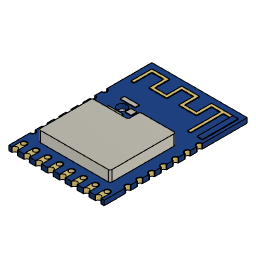
EMB1061_BLE4.2_BlueNRG-132 v2 (Autodesk Fusion 360 design; units mm, degrees)
Autodesk Fusion 360 part; units mm, degrees
sketch "Sketch1" plane through (0, 0, 0) normal (0, 0, 1) x (1, 0, 0)
  line L0 (16, 24) -> (0, 24)
  line L1 (1.5, 1.5) -> (1.5, 0)
  line L2 (0.5, 0) -> (0.5, 1.5)
  arc A0 (1.45, 0) -> (0.55, 0) centre (1, 0) ccw
  line L3 (2.5, 0) -> (2.5, 1.5)
  line L4 (3.5, 1.5) -> (3.5, 0)
  line L5 (3.5, 0) -> (3.45, 0)
  circle A1 centre (3, 1.5) radius 0.4
  arc A2 (3.45, 0) -> (2.55, 0) centre (3, 0) ccw
  line L6 (4.5, 0) -> (4.5, 1.5)
  line L7 (5.5, 1.5) -> (5.5, 0)
  circle A3 centre (5, 1.5) radius 0.4
  arc A4 (5.45, 0) -> (4.55, 0) centre (5, 0) ccw
  line L8 (6.5, 0) -> (6.5, 1.5)
  line L9 (7.5, 1.5) -> (7.5, 0)
  circle A5 centre (7, 1.5) radius 0.4
  arc A6 (7.45, 0) -> (6.55, 0) centre (7, 0) ccw
  line L10 (0.5, 0) -> (0.5, 1.5)
  line L11 (1.5, 1.5) -> (1.5, 0)
  circle A7 centre (1, 1.5) radius 0.4
  arc A8 (1.45, 0) -> (0.55, 0) centre (1, 0) ccw
  line L12 (9.5, 1.5) -> (9.5, 0)
  arc A9 (9.45, 0) -> (8.55, 0) centre (9, 0) ccw
  line L13 (8.5, 0) -> (8.5, 1.5)
  circle A10 centre (9, 1.5) radius 0.4
  line L14 (11.5, 1.5) -> (11.5, 0)
  arc A11 (11.45, 0) -> (10.55, 0) centre (11, 0) ccw
  line L15 (10.5, 0) -> (10.5, 1.5)
  circle A12 centre (11, 1.5) radius 0.4
  line L16 (13.5, 1.5) -> (13.5, 0)
  arc A13 (13.45, 0) -> (12.55, 0) centre (13, 0) ccw
  line L17 (12.5, 0) -> (12.5, 1.5)
  circle A14 centre (13, 1.5) radius 0.4
  line L18 (15.5, 1.5) -> (15.5, 0)
  arc A15 (15.45, 0) -> (14.55, 0) centre (15, 0) ccw
  line L19 (14.5, 0) -> (14.5, 1.5)
  circle A16 centre (15, 1.5) radius 0.4
  line L20 (1.5, 0) -> (1.45, 0)
  line L21 (0.55, 0) -> (0.5, 0)
  line L22 (1.5, 0) -> (1.45, 0)
  line L23 (0.55, 0) -> (0.5, 0)
  line L24 (5.5, 0) -> (5.45, 0)
  line L25 (4.55, 0) -> (4.5, 0)
  line L26 (3.45, 0) -> (4.55, 0)
  line L27 (7.5, 0) -> (7.45, 0)
  line L28 (6.55, 0) -> (6.5, 0)
  line L29 (5.45, 0) -> (6.55, 0)
  line L30 (7.45, 0) -> (8.55, 0)
  line L31 (9.45, 0) -> (10.55, 0)
  line L32 (11.45, 0) -> (12.55, 0)
  line L33 (13.45, 0) -> (14.55, 0)
  line L34 (15.45, 0) -> (16, 0)
  arc A17 (0, 3.6) -> (0, 4.4) centre (0, 4) ccw
  arc A18 (0, 5.6) -> (0, 6.4) centre (0, 6) ccw
  arc A19 (0, 7.6) -> (0, 8.4) centre (0, 8) ccw
  arc A20 (0, 9.6) -> (0, 10.4) centre (0, 10) ccw
  arc A21 (0, 11.6) -> (0, 12.4) centre (0, 12) ccw
  arc A22 (0, 13.6) -> (0, 14.4) centre (0, 14) ccw
  arc A23 (0, 15.6) -> (0, 16.4) centre (0, 16) ccw
  arc A24 (16, 6.4) -> (16, 5.6) centre (16, 6) ccw
  arc A25 (16, 16.4) -> (16, 15.6) centre (16, 16) ccw
  arc A26 (16, 4.4) -> (16, 3.6) centre (16, 4) ccw
  arc A27 (16, 10.4) -> (16, 9.6) centre (16, 10) ccw
  arc A28 (16, 8.4) -> (16, 7.6) centre (16, 8) ccw
  arc A29 (16, 14.4) -> (16, 13.6) centre (16, 14) ccw
  arc A30 (16, 12.4) -> (16, 11.6) centre (16, 12) ccw
  line L35 (0, 24) -> (0, 16.4)
  line L36 (0, 15.6) -> (0, 14.4)
  line L37 (0, 13.6) -> (0, 12.4)
  line L38 (0, 11.6) -> (0, 10.4)
  line L39 (0, 9.6) -> (0, 8.4)
  line L40 (0, 7.6) -> (0, 6.4)
  line L41 (0, 5.6) -> (0, 4.4)
  line L42 (0, 3.6) -> (0, 0)
  line L43 (0, 3.5) -> (0, 3.6)
  line L44 (0, 4.4) -> (0, 4.5)
  line L45 (16, 0) -> (16, 3.6)
  line L46 (16, 4.4) -> (16, 5.6)
  line L47 (16, 6.4) -> (16, 7.6)
  line L48 (16, 8.4) -> (16, 9.6)
  line L49 (16, 10.4) -> (16, 11.6)
  line L50 (16, 12.4) -> (16, 13.6)
  line L51 (16, 14.4) -> (16, 15.6)
  line L52 (16, 16.4) -> (16, 24)
  arc A31 (1.5, 1.5) -> (0.5, 1.5) centre (1, 1.5) ccw
  arc A32 (3.5, 1.5) -> (2.5, 1.5) centre (3, 1.5) ccw
  arc A33 (0, 3.5) -> (0, 4.5) centre (0, 4) ccw
  arc A34 (0, 5.5) -> (0, 6.5) centre (0, 6) ccw
  arc A35 (0, 7.5) -> (0, 8.5) centre (0, 8) ccw
  arc A36 (0, 9.5) -> (0, 10.5) centre (0, 10) ccw
  arc A37 (0, 11.5) -> (0, 12.5) centre (0, 12) ccw
  arc A38 (0, 13.5) -> (0, 14.5) centre (0, 14) ccw
  arc A39 (16, 16.5) -> (16, 15.5) centre (16, 16) ccw
  arc A40 (16, 14.5) -> (16, 13.5) centre (16, 14) ccw
  arc A41 (16, 12.5) -> (16, 11.5) centre (16, 12) ccw
  arc A42 (16, 10.5) -> (16, 9.5) centre (16, 10) ccw
  arc A43 (16, 6.5) -> (16, 5.5) centre (16, 6) ccw
  arc A44 (16, 4.5) -> (16, 3.5) centre (16, 4) ccw
  arc A45 (16, 8.5) -> (16, 7.5) centre (16, 8) ccw
  arc A46 (0, 15.5) -> (0, 16.5) centre (0, 16) ccw
  arc A47 (7.5, 1.5) -> (6.5, 1.5) centre (7, 1.5) ccw
  arc A48 (5.5, 1.5) -> (4.5, 1.5) centre (5, 1.5) ccw
  arc A49 (9.5, 1.5) -> (8.5, 1.5) centre (9, 1.5) ccw
  arc A50 (11.5, 1.5) -> (10.5, 1.5) centre (11, 1.5) ccw
  arc A51 (13.5, 1.5) -> (12.5, 1.5) centre (13, 1.5) ccw
  arc A52 (15.5, 1.5) -> (14.5, 1.5) centre (15, 1.5) ccw
  line L53 (0, 0) -> (0.55, 0)
  line L54 (1.45, 0) -> (2.55, 0)
  line L55 (13.5, 17) -> (13, 17)
  line L56 (13, 17) -> (13, 22.5)
  line L57 (13.5, 22.5) -> (13.5, 17)
  line L58 (1.5, 22.5) -> (1.5, 19.5)
  line L59 (1.5, 19.5) -> (1, 19.5)
  line L60 (1, 19.5) -> (1, 23)
  line L61 (1, 23) -> (4, 23)
  line L62 (4, 23) -> (4, 20.5)
  line L63 (3.5, 20) -> (3.5, 22.5)
  line L64 (4, 20.5) -> (6, 20.5)
  line L65 (6.5, 20) -> (3.5, 20)
  line L66 (6, 20.5) -> (6, 23)
  line L67 (6.5, 22.5) -> (6.5, 20)
  line L68 (9, 20.5) -> (11, 20.5)
  line L69 (8.5, 20) -> (8.5, 22.5)
  line L70 (9, 23) -> (9, 20.5)
  line L71 (8.5, 20) -> (11.5, 20)
  line L72 (11.5, 20) -> (11.5, 22.5)
  line L73 (11, 23) -> (11, 20.5)
  line L74 (14.6, 23) -> (11, 23)
  line L75 (11.5, 22.5) -> (13, 22.5)
  line L76 (9, 23) -> (6, 23)
  line L77 (1.5, 22.5) -> (3.5, 22.5)
  line L78 (6.5, 22.5) -> (8.5, 22.5)
  line L79 (13.5, 22.5) -> (14.6, 22.5)
  line L80 (14.6, 22.5) -> (14.6, 23)
  line L81 (2.3, 3) -> (13.7, 3)
  line L82 (14, 3.3) -> (14, 13.7)
  line L83 (13.7, 14) -> (8.3, 14)
  line L84 (2, 11.7) -> (2, 3.3)
  line L85 (2.3, 12) -> (7.7, 12)
  line L86 (8, 12.3) -> (8, 13.7)
  circle A53 centre (4, 15) radius 0.8
  line L87 (2.7, 16.7) -> (5.2, 16.7)
  line L88 (5.2, 16.7) -> (5.2, 16)
  line L89 (5.2, 16) -> (2.7, 16)
  line L90 (2.7, 16) -> (2.7, 16.7)
  line L91 (2.7, 14) -> (5.2, 14)
  line L92 (5.2, 14) -> (5.2, 13.3)
  line L93 (5.2, 13.3) -> (2.7, 13.3)
  line L94 (2.7, 13.3) -> (2.7, 14)
  line L95 (5, 15.5) -> (6, 15.5)
  line L96 (6, 15.5) -> (6, 14.5)
  line L97 (6, 14.5) -> (5, 14.5)
  line L98 (5, 14.5) -> (5, 15.5)
  arc A54 (8.3, 14) -> (8, 13.7) centre (8.3, 13.7) ccw
  arc A55 (14, 13.7) -> (13.7, 14) centre (13.7, 13.7) ccw
  arc A56 (13.7, 3) -> (14, 3.3) centre (13.7, 3.3) ccw
  arc A57 (2, 3.3) -> (2.3, 3) centre (2.3, 3.3) ccw
  arc A58 (2.3, 12) -> (2, 11.7) centre (2.3, 11.7) ccw
  arc A59 (7.7, 12) -> (8, 12.3) centre (7.7, 12.3) ccw
  line L99 (15.5, 23) -> (14.602, 23)
  line L100 (14.602, 23) -> (14.602, 17)
  line L101 (14.602, 17) -> (15.5, 17)
  line L102 (15.5, 17) -> (15.5, 23)
  dimension "d1" = 16
  dimension "d2" = 24
  dimension "d23" = 0.8
  dimension "d24" = 0.8
  dimension "d25" = 0.8
  dimension "d26" = 0.8
  dimension "d27" = 0.8
  dimension "d28" = 0.8
  dimension "d29" = 0.8
  dimension "d30" = 0.8
  dimension "d31" = 0.4
  dimension "d32" = 0.4
  dimension "d33" = 0.4
  dimension "d34" = 0.4
  dimension "d35" = 0.4
  dimension "d36" = 0.4
  dimension "d37" = 0.4
  dimension "d38" = 0.4
  dimension "d39" = 0.4
  dimension "d40" = 0.4
  dimension "d41" = 0.4
  dimension "d42" = 0.4
  dimension "d43" = 0.4
  dimension "d44" = 0.4
  dimension "d54" = 0.3
  constraint horizontal L53
  constraint vertical L45
  constraint horizontal L0
  constraint vertical L35
  constraint coincident L42.end L53.start
  constraint vertical L1
  constraint horizontal L20
  constraint vertical L2
  constraint coincident L1.end L53
  constraint coincident A0.start L53
  constraint vertical L4
  constraint horizontal L5
  constraint vertical L3
  constraint vertical L7
  constraint horizontal L24
  constraint vertical L6
  constraint vertical L9
  constraint horizontal L27
  constraint vertical L8
  constraint vertical L11
  constraint horizontal L22
  constraint vertical L10
  constraint vertical L12
  constraint vertical L13
  constraint vertical L14
  constraint vertical L15
  constraint vertical L16
  constraint vertical L17
  constraint vertical L18
  constraint vertical L19
  constraint collinear L20 L21
  constraint coincident A0.centre L20
  constraint collinear L26 L53
  constraint collinear L22 L23
  constraint coincident A0.centre L22
  constraint coincident A2.centre L5
  constraint collinear L24 L25
  constraint coincident A4.centre L24
  constraint collinear L26 L29
  constraint collinear L27 L28
  constraint coincident A6.centre L27
  constraint collinear L29 L30
  constraint collinear L30 L31
  constraint collinear L31 L32
  constraint collinear L32 L33
  constraint collinear L33 L34
  constraint coincident A17.centre L35
  constraint vertical L43
  constraint coincident L44.end L35
  constraint coincident A17.end L35
  constraint coincident A17.start L35
  constraint collinear L35 L36
  constraint collinear L36 L37
  constraint collinear L37 L38
  constraint collinear L38 L39
  constraint collinear L39 L40
  constraint collinear L40 L41
  constraint collinear L41 L42
  constraint collinear L43 L44
  constraint collinear L45 L46
  constraint collinear L46 L47
  constraint collinear L47 L48
  constraint collinear L48 L49
  constraint collinear L49 L50
  constraint collinear L50 L51
  constraint collinear L51 L52
  constraint concentric A7 A31
  constraint concentric A1 A32
  constraint concentric A3 A48
  constraint concentric A5 A47
  constraint concentric A10 A49
  constraint concentric A12 A50
  constraint concentric A14 A51
  constraint concentric A16 A52
  constraint concentric A26 A44
  constraint concentric A24 A43
  constraint concentric A27 A42
  constraint concentric A30 A41
  constraint concentric A29 A40
  constraint concentric A25 A39
  constraint concentric A23 A46
  constraint concentric A22 A38
  constraint concentric A21 A37
  constraint concentric A20 A36
  constraint concentric A19 A35
  constraint concentric A18 A34
  constraint concentric A17 A33
  constraint coincident L40 A34.end
  constraint coincident L41 A34.start
  constraint coincident L51 A39.end
  constraint coincident L52 A39.start
  constraint coincident L50 A40.end
  constraint coincident L51 A40.start
  constraint coincident L49 A41.end
  constraint coincident L50 A41.start
  constraint coincident L48 A42.end
  constraint coincident L49 A42.start
  constraint coincident L46 A43.end
  constraint coincident L47 A43.start
  constraint coincident L45 A44.end
  constraint coincident L46 A44.start
  constraint concentric A28 A45
  constraint coincident L47 A45.end
  constraint coincident L48 A45.start
  constraint coincident L35 A46.end
  constraint coincident L36 A46.start
  constraint collinear L53 L54
  constraint horizontal L55
  constraint horizontal L74
  constraint horizontal L77
  constraint vertical L58
  constraint horizontal L59
  constraint vertical L60
  constraint horizontal L61
  constraint vertical L62
  constraint vertical L63
  constraint horizontal L64
  constraint horizontal L65
  constraint vertical L66
  constraint vertical L67
  constraint coincident L66.end L74
  constraint horizontal L68
  constraint vertical L69
  constraint vertical L70
  constraint horizontal L71
  constraint vertical L72
  constraint vertical L73
  constraint collinear L74 L76
  constraint collinear L75 L77
  constraint collinear L77 L78
  constraint horizontal L79
  constraint vertical L80
  constraint horizontal L81
  constraint vertical L82
  constraint vertical L84
  constraint horizontal L85
  constraint vertical L86
  constraint horizontal L87
  constraint vertical L88
  constraint horizontal L89
  constraint vertical L90
  constraint horizontal L91
  constraint vertical L92
  constraint horizontal L93
  constraint vertical L94
  constraint horizontal L95
  constraint vertical L96
  constraint horizontal L97
  constraint vertical L98
  constraint tangent L86 A54
  constraint tangent L83 A54
  constraint tangent L82 A55
  constraint tangent L83 A55
  constraint equal A54 A55
  constraint tangent L81 A56
  constraint tangent L82 A56
  constraint equal A54 A56
  constraint tangent L81 A57
  constraint tangent L84 A57
  constraint equal A54 A57
  constraint tangent L85 A58
  constraint tangent L84 A58
  constraint equal A54 A58
  constraint tangent L85 A59
  constraint tangent L86 A59
  constraint equal A54 A59
  constraint horizontal L99
  constraint vertical L100
  constraint horizontal L101
  constraint vertical L102
  measures "d1" distance of L42.end L34.end
  measures "d2" distance of L42.end L0.end
  measures "d23" diameter of A7
  measures "d24" diameter of A1
  measures "d25" diameter of A3
  measures "d26" diameter of A10
  measures "d27" diameter of A5
  measures "d28" diameter of A12
  measures "d29" diameter of A14
  measures "d30" diameter of A16
  measures "d31" radius of A26
  measures "d32" radius of A24
  measures "d33" radius of A28
  measures "d34" radius of A27
  measures "d35" radius of A30
  measures "d36" radius of A29
  measures "d37" radius of A25
  measures "d38" radius of A23
  measures "d39" radius of A22
  measures "d40" radius of A21
  measures "d41" radius of A20
  measures "d42" radius of A19
  measures "d43" radius of A18
  measures "d44" radius of A17
  measures "d54" radius of A54
extrude "Extrude1" add sketch "Sketch1" along normal blind 0.8 contours L0 L1 L2 L3 L4 L6 L7 L8 L9 L10 L11 L12 L13 L14 L15 L16 L17 L18 L19 L26 L29 L30 L31 L32 L33 L34 L35 L36 L37 L38 L39 L40 L41 L42 L45 L46 L47 L48 L49 L50 L51 L52 A31 A32 A33 A34 A35 A36 A37 A38 A39 A40 A41 A42 A43 A44 A45 A46 A47 A48 A49 A50 A51 A52 L53 L54 | L55 L56 L57 L58 L59 L60 L61 L62 L63 L64 L65 L66 L67 L68 L69 L70 L71 L72 L73 L74 L75 L76 L77 L78 L79 L80 L100 | L80 L99 L100 L101 L102 | L81 L82 L83 L84 L85 L86 A54 A55 A56 A57 A58 A59 | L87 L88 L89 L90 | L91 L92 L93 L94 | L95 L96 L97 L98 makes body 1
extrude "Extrude2" add sketch "Sketch1" along normal blind 0.8 separate body contours A25 L51 L52 A39 | A23 L35 L36 A46 | A29 L50 L51 A40 | A22 L36 L37 A38 | A30 L49 L50 A41 | A21 L37 L38 A37 | A27 L48 L49 A42 | A20 L38 L39 A36 | A28 L47 L48 A45 | A19 L39 L40 A35 | A24 L46 L47 A43 | A18 L40 L41 A34 | A26 L45 L46 A44 | A17 L41 L42 L43 L44 A33 | L18 A15 L19 L33 L34 A52 | L1 L2 A0 L10 L11 A8 L20 L21 L22 L23 A31 L53 L54 | L16 A13 L17 L32 L33 A51 | L3 L4 L5 A2 L26 A32 L54 | L14 A11 L15 L31 L32 A50 | L6 L7 A4 L24 L25 L26 L29 A48 | L12 A9 L13 L30 L31 A49 | L8 L9 A6 L27 L28 L29 L30 A47 makes body 2 at (0.4998, 12.0125, 0.5333) makes body 3 at (0.3214, 4.383, 0.2667) makes body 4 at (15.6251, 10.3308, 0.5333) makes body 5 at (15.398, 1.4602, 0.5333) makes body 6 at (7.398, 1.4602, 0.5333) makes body 7 at (3.398, 1.4602, 0.5333) makes body 8 at (9.398, 1.4602, 0.5333) makes body 9 at (15.7393, 3.5734, 0.2667) makes body 10 at (15.6251, 12.3308, 0.5333) makes body 11 at (0.3214, 6.383, 0.2667) makes body 12 at (0.4998, 13.9875, 0.5333) makes body 13 at (0.4998, 10.0125, 0.5333) makes body 14 at (15.5442, 15.7944, 0.2667) makes body 15 at (15.829, 7.5302, 0.5333) makes body 16 at (13.398, 1.4602, 0.5333) makes body 17 at (5.398, 1.4602, 0.5333) makes body 18 at (1.398, 1.4602, 0.5333) makes body 19 at (11.398, 1.4602, 0.5333) makes body 20 at (15.7393, 5.5734, 0.2667) makes body 21 at (15.6251, 14.3308, 0.5333) makes body 22 at (0.4558, 8.2056, 0.2667) makes body 23 at (0.2607, 16.4266, 0.2667)
extrude "Extrude3" add sketch "Sketch1" along normal blind 0.8 and the other way blind -2.6 separate body contours L81 L82 L83 L84 L85 L86 A54 A55 A56 A57 A58 A59 makes body 24
extrude "Extrude4" add sketch "Sketch1" along normal blind 0.8 and the other way blind -0.9 separate body contours L55 L56 L57 L58 L59 L60 L61 L62 L63 L64 L65 L66 L67 L68 L69 L70 L71 L72 L73 L74 L75 L76 L77 L78 L79 L80 | L87 L88 L89 L90 | L91 L92 L93 L94 | L95 L96 L97 L98 | L99 L100 L101 L102 makes body 25 at (12.8667, 22.8333, 0.9) makes body 26 at (5.3333, 15.1667, 0.9) makes body 27 at (3.5333, 16.4667, 0.9) makes body 28 at (3.5333, 13.7667, 0.9) makes body 29 at (14.9013, 21, 0.9)
